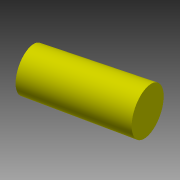
# Autodesk Inventor part: 32913_roller
Saved by Autodesk Inventor 2014 SP2 (Build 180246200, 246)
## iProperties
Created: 2018-11-17
Part Number: 32913_roller
Material: Generic
Catalog Web Link: www.cadenas.de
Description: BT1_001_101_roller-Tapered roller bearings, single row
Vendor: SKF
Document SubType Name: Modeling
Designer: psadmin
Manufacturer: SKF
Mass: 0.259207 g
Surface Area: 2.41856 cm^2
Volume: 0.259207 cm^3
Density: 1 g/cm^3
Appearance: PSOLRGB-255-255-0
Category: PARTsolutions
Company: SKF
Title: 32913_roller
Author: Cadenas PARTsolutions
Comments: Tapered roller bearings, single row
PSOL_IDENT_0: {$CADENAS_DATA\23d-libs\skf\bearings_units_and_housings\roller_bearings\tapered_roller_bearings\tape
PSOL_IDENT_1: red_roller_bearings_single_row\parts\bt1_001_101_roller.prj},178 {VTYP=3D},{NB=32913_roller},{LINA=3
PSOL_IDENT_2: 2913_roller},{NN=BT1_001_101_roller},{DATE=14.08.2018 07:35:10},{GEOMDATE=29.05.2018 10:30:25},{VERS
PSOL_IDENT_3: ION=},{LINEID=3110},{WBVAR=},{WBNUMERIC=}  {NB=32913_roller},{LINA=32913_roller},{KT=DUMMY},{DESIGNA
PSOL_IDENT_4: TION=32913},{DD=65.000},{D=90.000},{T=17.000},{DD1=78.8000},{D1=MIN},{B=17.000},{C=14.000},{C1=MIN},
PSOL_IDENT_5: {R12=1.0},{R34=1.0},{AA=16.53733},{PITCH=77.207},{DW=5.200},{LW=12.200},{RANGLE=1.600},{ALPHA=13.250
PSOL_IDENT_6: },{DDAMAX=71},{DDAMIN=73.0},{DAMIN=83},{DAMAX=83.0},{DBMIN=86},{CA=3},{CB=3.0},{RA=1.0},{RB=1.0},{LO
PSOL_IDENT_7: AD1=54.700},{LOAD2=80.000},{LOAD3=8.150},{SPEED1=5600},{SPEED2=6700},{EE=0.35},{Y=1.70},{Y0=0.9},{Y1=
PSOL_IDENT_8: 0},{X1=1},{X2=0.4},{X0=0.5},{Z=36},{II=1},{R1=0.00000231},{R2=10.9},{S1=0.009},{S2=2},{KZ=6},{KL=0.7
PSOL_IDENT_9: },{BF=2},{MASS=0.323},{PIM=PIM_BT1_001},{DESIGN=trb1},{HELP=0.000}
NN: BT1_001_101_roller
NT: Tapered roller bearings, single row
NB: 32913_roller
NBSYN: $DESIGNATION._roller
LINA: 32913_roller
DESIGNATION: 32913
DD: 65
D: 90
T: 17
DD1: 78.8
D1: 0
B: 17
C: 14
C1: 0
R12: 1
R34: 1
AA: 16.53733
PITCH: 77.207
DW: 5.2
LW: 12.2
RANGLE: 1.6
ALPHA: 13.25
DDAMAX: 71
DDAMIN: 73
DAMIN: 83
DAMAX: 83
DBMIN: 86
CA: 3
CB: 3
RA: 1
RB: 1
LOAD1: 54.7
LOAD2: 80
LOAD3: 8.15
SPEED1: 5600
SPEED2: 6700
EE: 0.35
Y: 1.7
Y0: 0.9
Y1: 0
X1: 1
X2: 0.4
X0: 0.5
Z: 36
II: 1
R1: 0.00000231
R2: 10.9
S1: 0.009
S2: 2
KZ: 6
KL: 0.7
BF: 2
MASS: 0.323
PIM: PIM_BT1_001
SUPPLIER: SKF
ARTICLENO: 32913_roller
BOMINFO: 32913_roller
CREATOR: CADENAS GmbH
Autodesk Inventor part; units mm, degrees
ref_plane "YZ Plane" through (0, 0, 0) normal (1, 0, 0) x (0, 1, 0)
ref_plane "XZ Plane" through (0, 0, 0) normal (0, 1, 0) x (-1, 0, 0)
ref_plane "XY Plane" through (0, 0, 0) normal (0, 0, 1) x (1, 0, 0)
sketch "Sketch_1" plane through (0, 0, 0) normal (0, 0, 1) x (1, 0, 0)
  line L0 (13.385, 40.0016) -> (1.5098, 37.2054)
  line L1 (1.5098, 37.2054) -> (0.9355, 39.6445)
  line L2 (0.9355, 39.6445) -> (12.7675, 42.6241)
  line L3 (12.7675, 42.6241) -> (13.385, 40.0016)
  line L4 (13.385, 40.0016) -> (1.5098, 37.2054)
  constraints: 10 end point
revolve "Revolution1" add sketch "Sketch_1" angle 360 about axis through (13.385, 40.0016, 0) along (0.9733793, 0.2292004, 0)
ref_plane "roller_XY" through (0, 38.6035, 0) normal (-1, 0, 0) x (0, 0, -1)
ref_plane "roller_YZ" through (0, 38.6035, 0) normal (0, 0, -1) x (0, -1, 0)
ref_plane "roller_ZX" through (0, 38.6035, 0) normal (0, -1, 0) x (-1, 0, 0)
body "Solid1"
